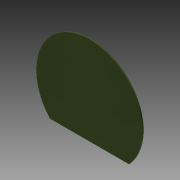
# Autodesk Inventor part: PCB
Saved by Autodesk Inventor 2015 (Build 190159000, 159)
## iProperties
Created: 2016-08-02
Part Number: PCB
Material: Generic
Document SubType Name: Modeling
Designer: James Yelland
Density: 1 g/cm^3
Appearance: Default
Author: James Yelland
Autodesk Inventor part; units mm, degrees
ref_plane "YZ Plane" through (0, 0, 0) normal (1, 0, 0) x (0, 1, 0)
ref_plane "XZ Plane" through (0, 0, 0) normal (0, 1, 0) x (-1, 0, 0)
ref_plane "XY Plane" through (0, 0, 0) normal (0, 0, 1) x (1, 0, 0)
sketch "Sketch1" plane through (0, 0, 0) normal (0, 1, 0) x (-1, 0, 0)
  line L0 (0, -60) -> (-67.082, -60)
  line L1 (0, -60) -> (67.082, -60)
  arc A0 (67.082, -60) -> (-67.082, -60) centre (0, 0) ccw
  line L2 (67.082, -60) -> (-67.082, -60)
  constraints: 6 end point, 2 point on circle, 1 centre point, 1 horizontal, 1 point on line
extrude "Extrusion1" add sketch "Sketch1" along normal blind 2
body "Solid1"
